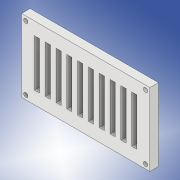
# Autodesk Inventor part: HA006
Saved by Autodesk Inventor 2017 SP1 (Build 210196100, 196)
## iProperties
Created: 2017-06-25
Part Number: HA006
Material: ABS Plastic
Document SubType Name: Modeling
Designer: Zach
Density: 1.06 g/cm^3
Appearance: CR White
Author: Zach
Autodesk Inventor part; units mm, degrees
ref_plane "YZ Plane" through (0, 0, 0) normal (1, 0, 0) x (0, 1, 0)
ref_plane "XZ Plane" through (0, 0, 0) normal (0, 1, 0) x (-1, 0, 0)
ref_plane "XY Plane" through (0, 0, 0) normal (0, 0, 1) x (1, 0, 0)
sketch "Sketch1" plane through (0, 0, 0) normal (0, 0, 1) x (1, 0, 0)
  line L0 (0, 0) -> (150, 0)
  line L1 (150, 0) -> (150, 85)
  line L2 (150, 85) -> (0, 85)
  line L3 (0, 85) -> (0, 0)
  dimension "d0" = 150
  dimension "d1" = 85
  constraints: 8 end point, 2 parallel, 1 horizontal, 1 perpendicular
  measures "d0" distance of L2.end L1.end
  measures "d1" distance of L1.end L0.end
extrude "Extrusion1" add sketch "Sketch1" along normal blind 10
sketch "Sketch2" plane through (0, 0, 10) normal (0, 0, 1) x (1, 0, 0)
  line L0 (0, 0) -> (150, 0) construction
  line L1 (150, 0) -> (150, 85) construction
  line L2 (150, 85) -> (0, 85) construction
  line L3 (0, 85) -> (0, 0) construction
  line L4 (5, 80) -> (145, 80) construction
  line L5 (145, 80) -> (145, 5) construction
  line L6 (145, 5) -> (5, 5) construction
  line L7 (5, 5) -> (5, 80) construction
  line L8 (10, 75) -> (140, 75) construction
  line L9 (140, 75) -> (140, 10) construction
  line L10 (140, 10) -> (10, 10) construction
  line L11 (10, 10) -> (10, 75) construction
  circle A0 centre (5, 80) radius 2.5
  circle A1 centre (145, 80) radius 2.5
  circle A2 centre (145, 5) radius 2.5
  circle A3 centre (5, 5) radius 2.5
  line L12 (15, 70) -> (21, 70)
  line L13 (21, 70) -> (21, 15)
  line L14 (21, 15) -> (15, 15)
  line L15 (15, 15) -> (15, 70)
  line L16 (15, 70) -> (135, 70) construction
  line L17 (135, 70) -> (135, 15) construction
  line L18 (135, 15) -> (15, 15) construction
  line L19 (15, 15) -> (15, 70) construction
  line L20 (33.65, 70) -> (33.65, 15)
  line L21 (27.65, 70) -> (33.65, 70)
  line L22 (27.65, 15) -> (27.65, 70)
  line L23 (27.65, 15) -> (27.65, 70) construction
  line L24 (33.65, 15) -> (27.65, 15)
  line L25 (46.3, 70) -> (46.3, 15)
  line L26 (40.3, 70) -> (46.3, 70)
  line L27 (40.3, 15) -> (40.3, 70)
  line L28 (40.3, 15) -> (40.3, 70) construction
  line L29 (46.3, 15) -> (40.3, 15)
  line L30 (58.95, 70) -> (58.95, 15)
  line L31 (52.95, 70) -> (58.95, 70)
  line L32 (52.95, 15) -> (52.95, 70)
  line L33 (52.95, 15) -> (52.95, 70) construction
  line L34 (58.95, 15) -> (52.95, 15)
  line L35 (71.6, 70) -> (71.6, 15)
  line L36 (65.6, 70) -> (71.6, 70)
  line L37 (65.6, 15) -> (65.6, 70)
  line L38 (65.6, 15) -> (65.6, 70) construction
  line L39 (71.6, 15) -> (65.6, 15)
  line L40 (84.25, 70) -> (84.25, 15)
  line L41 (78.25, 70) -> (84.25, 70)
  line L42 (78.25, 15) -> (78.25, 70)
  line L43 (78.25, 15) -> (78.25, 70) construction
  line L44 (84.25, 15) -> (78.25, 15)
  line L45 (96.9, 70) -> (96.9, 15)
  line L46 (90.9, 70) -> (96.9, 70)
  line L47 (90.9, 15) -> (90.9, 70)
  line L48 (90.9, 15) -> (90.9, 70) construction
  line L49 (96.9, 15) -> (90.9, 15)
  line L50 (109.55, 70) -> (109.55, 15)
  line L51 (103.55, 70) -> (109.55, 70)
  line L52 (103.55, 15) -> (103.55, 70)
  line L53 (103.55, 15) -> (103.55, 70) construction
  line L54 (109.55, 15) -> (103.55, 15)
  line L55 (122.2, 70) -> (122.2, 15)
  line L56 (116.2, 70) -> (122.2, 70)
  line L57 (116.2, 15) -> (116.2, 70)
  line L58 (116.2, 15) -> (116.2, 70) construction
  line L59 (122.2, 15) -> (116.2, 15)
  line L60 (134.85, 70) -> (134.85, 15)
  line L61 (128.85, 70) -> (134.85, 70)
  line L62 (128.85, 15) -> (128.85, 70)
  line L63 (128.85, 15) -> (128.85, 70) construction
  line L64 (134.85, 15) -> (128.85, 15)
  dimension "d4" = 5
  dimension "d5" = 10
  dimension "d6" = 5
  dimension "d7" = 5
  dimension "d8" = 5
  dimension "d9" = 5
  dimension "d10" = 6
  dimension "d11" = 15
  dimension "d14" = 12.65
  constraints: 122 end point, 4 centre point, 4 coincident, 2 horizontal, 2 parallel, 1 perpendicular, 1 point on line, 99 other
  measures "d4" distance between parallel lines of L2 L4
  measures "d5" distance between parallel lines of L2 L8
  measures "d6" diameter of A0
  measures "d7" diameter of A1
  measures "d8" diameter of A2
  measures "d9" diameter of A3
  measures "d10" distance of L14.end L13.end
  measures "d11" distance between parallel lines of L2 L16
  measures "d14" distance of L12.end L20.start
extrude "Extrusion2" cut sketch "Sketch2" against normal through all
body "Solid1"
